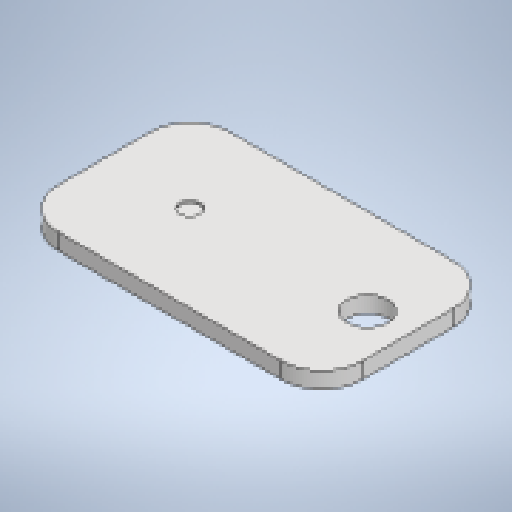
# Autodesk Inventor part: PNS 1783 leg floor plate
Saved by Autodesk Inventor 2025.1 (Build 291241020, 241B)
## iProperties
Created: 2025-02-20
Part Number: PNS 1783 leg floor plate
Material: Steel
Document SubType Name: Sheet Metal
Designer: admin
Mass: 1125.27 g
Surface Area: 340.013 cm^2
Volume: 143.346 cm^3
Density: 7.85 g/cm^3
Sheet Metal Rule: AISI304 3mm Die 32
Sheet Metal Width: 85.000 mm
Sheet Metal Length: 150.000 mm
Sheet Metal Area: 12750.000 mm^2
Appearance: Default
Flat Pattern Width: 8.5 cm
Flat Pattern Length: 15 cm
Flat Pattern Area: 127.5 cm^2
Author: user
Autodesk Inventor part; units mm, degrees
ref_plane "YZ Plane" through (0, 0, 0) normal (1, 0, 0) x (0, 1, 0)
ref_plane "XZ Plane" through (0, 0, 0) normal (0, 1, 0) x (-1, 0, 0)
ref_plane "XY Plane" through (0, 0, 0) normal (0, 0, 1) x (1, 0, 0)
sketch "Sketch1" plane through (0, 0, 0) normal (0, 0, 1) x (1, 0, 0)
  line L0 (-75, -42.5) -> (75, -42.5)
  line L1 (75, -42.5) -> (75, 42.5)
  line L2 (75, 42.5) -> (-75, 42.5)
  line L3 (-75, 42.5) -> (-75, -42.5)
  line L4 (-75, -42.5) -> (75, 42.5) construction
  line L5 (75, -42.5) -> (-75, 42.5) construction
  circle A0 centre (55, -22.5) radius 10
  circle A1 centre (55, 22.5) radius 10
  line L6 (0, 0) -> (75, 0) construction
  circle A2 centre (55, 0) radius 10
  dimension "d0" = 150
  dimension "d1" = 85
  dimension "d23" = 20
  dimension "d25" = 20
  dimension "d26" = 20
  measures "d0" distance of L2.end L1.end
  measures "d1" distance of L1.end L0.end
  measures "d23" diameter of A0
  measures "d25" distance from line of L1 A0.centre
  measures "d26" distance from line of A0.centre L0
extrude "Plate1" add sketch "Sketch1" along normal blind 8 contours L3 L2 L1 L0 | A0 | A1
fillet "Corner Round1" radius 5 4 edges at (75, -42.5, 4) (-75, -42.5, 4) (-75, 42.5, 4) (75, 42.5, 4)
sketch "Sketch5" plane through (0, 0, 8) normal (0, 0, 1) x (1, 0, 0)
  line L0 (70, -42.5) -> (-70, -42.5) projected
  line L1 (-75, -37.5) -> (-75, 37.5) projected
  line L2 (-70, 42.5) -> (70, 42.5) projected
  circle A0 centre (-32.5, 0) radius 42.5
  circle A1 centre (-32.5, 0) radius 5
  point P0 (0, 0)
  dimension "d27" = 10
  constraints: 3 tangent, 2 centre point, 1 coincident
  measures "d27" diameter of A1
extrude "Extrusion2" cut sketch "Sketch5" against normal blind 1 contours A1
equation "\"d26\" = d25"
equation "\"d2\" = Thickness"
equation "\"BendReliefWidth\" = Thickness"
equation "\"BendReliefDepth\" = 0.5 * Thickness"
equation "\"CornerReliefSize\" = 4 * Thickness"
equation "\"MinimumRemnant\" = 2 * Thickness"
equation "\"TransitionRadius\" = BendRadius"
equation "\"JacobiRadiusSize\" = BendRadius"
equation "\"GapSize\" = Thickness"
equation "\"Thickness\" = 8"
equation "\"BendRadius\" = 5"
body "Solid1"
